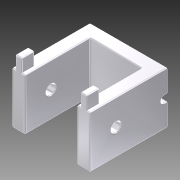
# Autodesk Inventor part: Tension_Housing
Saved by Autodesk Inventor 2012 (Build 160160000, 160)
## iProperties
Created: 2012-10-03
Part Number: Tension_Housing
Material: Default
Document SubType Name: Modeling
Designer: agmlego
Density: 1 g/cm^3
Author: agmlego
Autodesk Inventor part; units mm, degrees
ref_plane "YZ Plane" through (0, 0, 0) normal (1, 0, 0) x (0, 1, 0)
ref_plane "XZ Plane" through (0, 0, 0) normal (0, 1, 0) x (-1, 0, 0)
ref_plane "XY Plane" through (0, 0, 0) normal (0, 0, 1) x (1, 0, 0)
sketch "Sketch1" plane through (0, 0, 0) normal (0, 0, 1) x (1, 0, 0)
  line L0 (-15, 15) -> (15, 15)
  line L1 (15, 15) -> (15, -15)
  line L2 (-15, -15) -> (-15, 15)
  line L3 (-10, 10) -> (10, 10)
  line L4 (10, 10) -> (10, -15)
  line L5 (-10, -15) -> (-10, 10)
  line L6 (15, -15) -> (10, -15)
  line L7 (-10, -15) -> (-15, -15)
  point P0 (0, 0)
  dimension "d3" = 30
  dimension "d4" = 15
  dimension "d5" = 15
  dimension "d6" = 5
  dimension "d7" = 5
  constraints: 16 end point, 4 parallel, 3 equal length, 2 horizontal, 2 perpendicular
  measures "d3" distance of L0.start L0.end
  measures "d4" distance from line of L0 point (0, 0)
  measures "d5" distance from line of L2 point (0, 0)
  measures "d6" distance between parallel lines of L0 L3
  measures "d7" distance between parallel lines of L5 L2
extrude "Extrusion1" add sketch "Sketch1" along normal blind 20
sketch "Sketch2" plane through (0, 0, 20) normal (0, 0, 1) x (1, 0, 0)
  line L0 (-15, -15) -> (-15, 15) projected
  line L1 (-10, -15) -> (-15, -15) projected
  line L2 (10, -15) -> (10, 10) projected
  line L3 (15, -15) -> (10, -15) projected
  line L4 (-13.75, -10) -> (-11.25, -10)
  line L5 (-11.25, -10) -> (-11.25, -15)
  line L6 (-11.25, -15) -> (-13.75, -15)
  line L7 (-13.75, -15) -> (-13.75, -10)
  line L8 (11.25, -10) -> (13.75, -10)
  line L9 (13.75, -10) -> (13.75, -15)
  line L10 (13.75, -15) -> (11.25, -15)
  line L11 (11.25, -15) -> (11.25, -10)
  point P0 (0, 0)
  dimension "d10" = 2.5
  dimension "d11" = 1.25
  dimension "d12" = 1.25
  dimension "d13" = 5
  constraints: 16 end point, 4 parallel, 2 equal length, 2 horizontal, 2 perpendicular, 2 point on line
  measures "d10" distance of L5.end L6.end
  measures "d11" distance between parallel lines of L0 L7
  measures "d12" distance between parallel lines of L2 L11
  measures "d13" distance of L6.end L4.start
extrude "Extrusion2" add sketch "Sketch2" along normal blind 5
sketch "Sketch3" plane through (-15, 15, 0) normal (0, 1, 0) x (1, 0, 0)
  line L0 (0, -20) -> (30, -20) projected
  line L1 (30, 0) -> (30, -20) projected
  line L2 (0, 0) -> (0, -20) projected
  line L3 (0, -8.75) -> (30, -8.75)
  line L4 (30, -8.75) -> (30, -11.25)
  line L5 (30, -11.25) -> (0, -11.25)
  line L6 (0, -11.25) -> (0, -8.75) construction
  line L7 (15, 0) -> (15, -8.75) construction
  line L8 (15, -11.25) -> (15, -20) construction
  line L9 (0, -8.75) -> (0, -11.25)
  dimension "d16" = 2.5
  constraints: 14 end point, 3 equal length, 3 midpoint, 2 point on line, 1 collinear, 1 horizontal, 1 perpendicular
  measures "d16" distance of L5.end L3.start
extrude "Extrusion3" cut sketch "Sketch3" against normal blind 2.5 contours L2 L3 L1 L5
hole "Hole2" at (15, -5, 10) direction (-1, 0, 0) diameter 3.4 end through all clearance for "Flat Head Machine Screw" size "M3" standard "Ansi Metric M Profile"
fillet "Fillet6" radius 1.25 2 edges at (0, 12.5, 11.25) (0, 12.5, 8.75)
fillet "Fillet7" radius 0.5 60 edges at (15, 0, 20) (15, 15, 15.625) (15, 14.375, 8.75) (15, 14.375, 11.25) (15, 12.8661, 9.1161) (15, 12.5, 10) (15, 12.8661, 10.8839) (15, 15, 4.375) (15, 0, 0) (15, -15, 10) (15, -5, 11.7) (0, 15, 20) (0, 15, 11.25) (0, 15, 8.75) (0, 15, 0) (-15, 15, 4.375) (-15, 14.375, 11.25) (-15, 14.375, 8.75) (-15, 12.8661, 9.1161) (-15, 12.5, 10) (-15, 12.8661, 10.8839) (-15, 15, 15.625) (13.75, -10, 22.5) (13.75, -12.5, 25) (12.5, -10, 25) (11.25, -12.5, 25) (11.25, -10, 22.5) (11.25, -15, 22.5) (12.5, -15, 25) (13.75, -15, 22.5) (14.375, -15, 20) (10.625, -15, 20) (10, -2.5, 20) (10, -15, 10) (12.5, -15, 0) (10, -2.5, 0) (10, -5, 11.7) (0, 10, 20) (-10, -2.5, 20) (-10, 10, 10) (10, 10, 10) (0, 10, 0) (-10, -2.5, 0) (-10, -5, 11.7) (-10, -15, 10) (-15, -15, 10) (-12.5, -15, 0) (-15, 0, 0) (-15, -5, 11.7) (-10.625, -15, 20) (-14.375, -15, 20) (-11.25, -10, 22.5) (-13.75, -10, 22.5) (-13.75, -15, 22.5) (-11.25, -15, 22.5) (-11.25, -12.5, 25) (-13.75, -12.5, 25) (-12.5, -10, 25) (-12.5, -15, 25) (-15, 0, 20)
equation "\"d4\" = 0.5 * d3"
equation "\"d5\" = d4"
equation "\"d7\" = d6"
body "Solid1"
